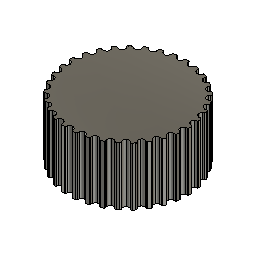
gear_33z (Autodesk Fusion 360 design; units mm, degrees)
Autodesk Fusion 360 part; units mm, degrees
sketch "Sketch1" plane through (0, 0, 0) normal (0, 0, 1) x (1, 0, 0) in component "gt2 pulley"
  circle A0 centre (0, 0) radius 10.5042 construction
  circle A1 centre (0, 0) radius 9.5002 construction
  line L0 (0, 0) -> (0, 10.5042) construction
  line L1 (0, 0) -> (0.9985, 10.4567) construction
  line L2 (0, 0) -> (1.4096, 10.4092) construction
  circle A2 centre (0, 0) radius 10.2502 construction
  arc A3 (0.3769, 10.1055) -> (0.4323, 9.8253) centre (1.3755, 10.1575) ccw
  circle A4 centre (0, 0) radius 10.1002 construction
  arc A5 (0.2304, 10.2476) -> (0, 10.2502) centre (0, 0) ccw
  arc A6 (0.3769, 10.1055) -> (0.2304, 10.2476) centre (0.2271, 10.0977) ccw
  arc A7 (0.4323, 9.8253) -> (0.9031, 9.4572) centre (0.9558, 10.0097) ccw
  arc A8 (0, 10.2502) -> (-0.2304, 10.2476) centre (0, 0) ccw
  arc A9 (-0.2304, 10.2476) -> (-0.3769, 10.1055) centre (-0.2271, 10.0977) ccw
  arc A10 (-0.4323, 9.8253) -> (-0.3769, 10.1055) centre (-1.3755, 10.1575) ccw
  arc A11 (-0.9027, 9.4572) -> (-0.4323, 9.8253) centre (-0.9558, 10.0097) ccw
  arc A12 (0.9031, 9.4572) -> (-0.9031, 9.4572) centre (0, 0) ccw
  point P0 (1.3755, 10.1575)
  point P1 (0, 10.2502)
  dimension "d18" = 21.0085
  dimension "d19" = 5.455
  dimension "d22" = 1.004
  dimension "d24" = 0.75
  dimension "d26" = 1
  dimension "d27" = 0.15
  dimension "d28" = 0.15
  dimension "d47" = 0.555
  dimension "d52" = 3.812
  constraint coincident A0.centre A1.centre
  constraint coincident A0 L0.end
  constraint vertical L0
  constraint coincident A0 L1.end
  constraint coincident A0 L2.end
  constraint concentric A1 A2
  constraint coincident A1 A7.end
  constraint coincident L1 A7.end
  constraint coincident A2 P0
  constraint coincident L2 P0
  constraint coincident P0 A3.centre
  constraint coincident A2 P1
  constraint coincident L0 P1
  constraint concentric A2 A4
  constraint coincident P1 A5.end
  constraint coincident A4 A6.centre
  constraint coincident A3.start A6.start
  constraint tangent A3 A6
  constraint tangent A3 A7
  constraint symmetric L0 A7.end A12.end
  constraint symmetric L0 A3.start A9.end
  constraint symmetric L0 A3.end A10.start
  constraint symmetric L0 A3 A10
  constraint symmetric L0 A5.start A8.end
  constraint symmetric L0 P1 A5.end
  constraint symmetric L0 A5 A8
  constraint symmetric L0 A6 A9
  constraint symmetric L0 A7 A11
  constraint coincident A1 A11.start
  constraint tangent A1 A7
  constraint coincident L1 A7.centre
  measures "d18" diameter of A0
  measures "d19" angle of L0 L1
  measures "d22" distance of A0 A1
  measures "d24" distance of A1 A2
  measures "d26" radius of A3
  measures "d27" distance of A2 A4
  measures "d28" radius of A6
  measures "d47" radius of A7
extrude "Extrude1" add sketch "Sketch1" along normal blind 10 makes body 1
pattern_circular "C-Pattern1" count 33 over 360 about axis through (0, 0, 1.75) along (0, 0, 1) of bodies 1 makes body 2 at (-2.4828, 9.1701, 6.6667) makes body 3 at (-2.8687, 9.0568, 3.3333) makes body 4 at (-5.2203, 7.9374, 6.6667) makes body 5 at (-6.0293, 7.3418, 3.3333) makes body 6 at (-7.7964, 5.4287, 6.6667) makes body 7 at (-8.8382, 3.4844, 3.3333) makes body 8 at (-9.2082, 2.3374, 3.3333) makes body 9 at (-9.43, 1.1528, 3.3333) makes body 10 at (-9.4778, -0.6526, 3.3333) makes body 11 at (-8.9444, -3.2018, 6.6667) makes body 12 at (-8.1768, -4.8367, 6.6667) makes body 13 at (-7.6204, -5.6731, 3.3333) makes body 14 at (-5.7935, -7.5293, 6.6667) makes body 15 at (-4.966, -8.0989, 3.3333) makes body 16 at (-3.3436, -8.8924, 3.3333) makes body 17 at (-1.6002, -9.3645, 3.3333) makes body 18 at (1.0029, -9.4471, 6.6667) makes body 19 at (2.7726, -9.0866, 6.6667) makes body 20 at (4.4422, -8.3977, 6.6667) makes body 21 at (6.4088, -7.013, 6.6667) makes body 22 at (7.6202, -5.6734, 6.6667) makes body 23 at (8.2771, -4.663, 6.6667) makes body 24 at (8.7232, -3.7629, 3.3333) makes body 25 at (9.2777, -2.044, 3.3333) makes body 26 at (9.4969, -0.2512, 3.3333) makes body 27 at (9.0415, 2.9163, 6.6667) makes body 28 at (8.3262, 4.5747, 6.6667) makes body 29 at (8.1251, 4.9231, 3.3333) makes body 30 at (7.0466, 6.3718, 3.3333) makes body 31 at (4.5312, 8.35, 6.6667) makes body 32 at (4.1737, 8.5343, 3.3333) makes body 33 at (1.6993, 9.347, 6.6667)
sketch "Sketch2" plane through (0, 0, 10) normal (0, 0, 1) x (-1, 0, 0)
  arc A0 (-2.2826, -9.8515) -> (-2.1656, -10.0188) centre (-2.134, -9.8722) ccw
  arc A1 (-2.1656, -10.0188) -> (-1.7131, -10.1061) centre (0, 0) ccw
  arc A2 (-1.7131, -10.1061) -> (-1.5424, -9.9942) centre (-1.688, -9.9582) ccw
  arc A3 (-1.4349, -9.7296) -> (-1.5424, -9.9942) centre (-0.5716, -10.2343) ccw
  arc A4 (-0.9034, -9.4572) -> (-1.4349, -9.7296) centre (-0.9558, -10.0097) ccw
  arc A5 (-2.6765, -9.1154) -> (-0.9034, -9.4572) centre (0, 0) ccw
  arc A6 (-2.284, -9.566) -> (-2.6765, -9.1154) centre (-2.8329, -9.6479) ccw
  arc A7 (-2.2826, -9.8515) -> (-2.284, -9.566) centre (-3.273, -9.7136) ccw
  circle A8 centre (0, 0) radius 9.5002
  constraint concentric A1 A8
extrude "Extrude2" add sketch "Sketch2" against normal blind 10 contours A5 A8 bodies 1 2 3 4 5 6 7 8 9 10 11 12 13 14 15 16 17 18 19 20 21 22 23 24 25 26 27 28 29 30 31 32 33
extrude "Extrude4" [suppressed] in component "gt2 pulley"
pattern_circular "C-Pattern7" [suppressed] in component "gt2 pulley"
extrude "Extrude3" [suppressed] in component "gt2 pulley"
pattern_circular "C-Pattern6" [suppressed] in component "gt2 pulley"
extrude "Extrude2'" [suppressed] in component "gt2 pulley"
pattern_circular "C-Pattern5" [suppressed] in component "gt2 pulley"
extrude "Extrude1'" [suppressed] in component "gt2 pulley"
pattern_circular "C-Pattern4" [suppressed] in component "gt2 pulley"
pattern_circular "C-Pattern3" [suppressed] in component "gt2 pulley"
pattern_circular "C-Pattern2" [suppressed] in component "gt2 pulley"
pattern_circular "C-Pattern1'" [suppressed] in component "gt2 pulley"
copy_body "Body->Comp1" [suppressed] in component "Component"
copy_body "Body->Comp2" [suppressed] in component "Component'"
copy_body "Body->Comp3" [suppressed] in component "Component''"
copy_body "Body->Comp4" [suppressed] in component "Component'''"
copy_body "Body->Comp5" [suppressed] in component "Component''''"
copy_body "Body->Comp6" [suppressed] in component "Component'''''"
copy_body "Body->Comp7" [suppressed] in component "Component''''''"
copy_body "Body->Comp8" [suppressed] in component "Component'''''''"
copy_body "Body->Comp9" [suppressed] in component "Component''''''''"
copy_body "Body->Comp10" [suppressed] in component "Component'''''''''"
copy_body "Body->Comp11" [suppressed] in component "Component''''''''''"
copy_body "Body->Comp12" [suppressed] in component "Component'''''''''''"
copy_body "Body->Comp13" [suppressed] in component "Component''''''''''''"
copy_body "Body->Comp14" [suppressed] in component "Component'''''''''''''"
copy_body "Body->Comp15" [suppressed] in component "Component''''''''''''''"
copy_body "Body->Comp16" [suppressed] in component "Component'''''''''''''''"
copy_body "Body->Comp17" [suppressed] in component "Component''''''''''''''''"
copy_body "Body->Comp18" [suppressed] in component "Component'''''''''''''''''"
copy_body "Body->Comp19" [suppressed] in component "Component''''''''''''''''''"
copy_body "Body->Comp20" [suppressed] in component "Component'''''''''''''''''''"
component "gt2 pulley" placed x (1, 0, 0) y (0, 1, 0) z (0, 0, 1) at (0, 0, 0)
equation "NumTeeth = 33" comment "min 20"
equation "ToothPitch = 2 mm"
equation "PullyDia = NumTeeth * ToothPitch / PI"
equation "ToothAng = ( ( 360 / NumTeeth ) * 1 deg )"
equation "TransOffsetAngle = ToothAng * 0.2"
equation "Sholulder_Radius = 0.15 mm"
equation "Root_Radius = 0.555 mm"
equation "TransRadius = 1 mm"
equation "ToolHeight = 0.75 mm"
equation "PLD = 0.254 mm"
equation "d18 = PullyDia"
equation "d19 = ToothAng / 2"
equation "d22 = PLD + ToolHeight"
equation "d24 = ToolHeight"
equation "d26 = TransRadius"
equation "d27 = Sholulder_Radius"
equation "d31 = NumTeeth"
equation "d33 = NumTeeth"
equation "d35 = NumTeeth"
equation "d37 = NumTeeth"
equation "d41 = NumTeeth"
equation "d45 = NumTeeth"
equation "d47 = Root_Radius"
equation "d50 = NumTeeth"
